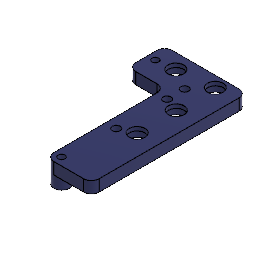
ZumoButtonAdapter (Autodesk Fusion 360 design; units mm, degrees)
Autodesk Fusion 360 part; units mm, degrees
sketch "Sketch1" plane through (17.2307, 33.6297, 85.118) normal (0, 0, 1) x (-0.000239, -1, 0)
  line L0 (5.7619, -33.0186) -> (14.2709, -33.0166)
  line L1 (14.2709, -33.0166) -> (14.2707, -32.1784)
  arc A0 (15.0833, -31.3654) -> (14.2707, -32.1784) centre (15.0835, -32.1782) ccw
  line L2 (15.0833, -31.3654) -> (20.4427, -31.3641)
  arc A1 (21.2557, -32.1767) -> (20.4427, -31.3641) centre (20.4429, -32.1769) ccw
  line L3 (21.2557, -32.1767) -> (21.2559, -33.0149)
  line L4 (21.2559, -33.0149) -> (36.4451, -33.0113)
  arc A2 (36.4451, -33.0113) -> (37.2577, -32.1983) centre (36.4449, -32.1985) ccw
  line L5 (37.2577, -32.1983) -> (37.2544, -18.2791)
  line L6 (37.2544, -18.2791) -> (35.9841, -17.0094)
  line L7 (35.9841, -17.0094) -> (35.9813, -5.3254)
  line L8 (35.9813, -5.3254) -> (37.251, -4.0551)
  line L9 (37.251, -4.0551) -> (37.249, 4.0729)
  line L10 (37.249, 4.0729) -> (35.4706, 5.8505)
  line L11 (35.4706, 5.8505) -> (35.4684, 14.9945)
  line L12 (35.4684, 14.9945) -> (37.246, 16.7729)
  line L13 (37.246, 16.7729) -> (37.2423, 32.2161)
  arc A3 (37.2423, 32.2161) -> (36.4293, 33.0287) centre (36.4295, 32.2159) ccw
  line L14 (36.4293, 33.0287) -> (21.2401, 33.0251)
  line L15 (21.2401, 33.0251) -> (21.2403, 32.1869)
  arc A4 (20.4277, 31.3739) -> (21.2403, 32.1869) centre (20.4275, 32.1867) ccw
  line L16 (20.4277, 31.3739) -> (15.0683, 31.3726)
  arc A5 (14.2553, 32.1852) -> (15.0683, 31.3726) centre (15.0681, 32.1854) ccw
  line L17 (14.2553, 32.1852) -> (14.2551, 33.0234)
  line L18 (14.2551, 33.0234) -> (5.7461, 33.0214)
  arc A6 (-0.6054, 39.3699) -> (5.7461, 33.0214) centre (5.7446, 39.3714) ccw
  line L19 (-0.6054, 39.3699) -> (-0.6071, 46.1771)
  arc A7 (-0.6071, 46.1771) -> (-1.4201, 46.9897) centre (-1.4199, 46.1769) ccw
  line L20 (-1.4201, 46.9897) -> (-11.2245, 46.9873)
  arc A8 (-11.2245, 46.9873) -> (-12.0371, 46.1743) centre (-11.2243, 46.1745) ccw
  line L21 (-12.0371, 46.1743) -> (-12.0354, 39.3671)
  arc A9 (-18.3839, 33.0156) -> (-12.0354, 39.3671) centre (-18.3854, 39.3656) ccw
  line L22 (-18.3839, 33.0156) -> (-22.0161, 33.0147)
  arc A10 (-22.8291, 33.8273) -> (-22.0161, 33.0147) centre (-22.0163, 33.8275) ccw
  line L23 (-22.8291, 33.8273) -> (-22.8302, 38.6025)
  line L24 (-22.8302, 38.6025) -> (-37.6892, 38.599)
  line L25 (-37.6892, 38.599) -> (-37.6881, 33.8238)
  arc A11 (-38.5007, 33.0108) -> (-37.6881, 33.8238) centre (-38.5009, 33.8236) ccw
  line L26 (-38.5007, 33.0108) -> (-44.7491, 33.0093)
  arc A12 (-44.7491, 33.0093) -> (-45.5617, 32.1963) centre (-44.7489, 32.1965) ccw
  line L27 (-45.5617, 32.1963) -> (-45.5463, -32.2181)
  arc A13 (-45.5463, -32.2181) -> (-44.7333, -33.0307) centre (-44.7335, -32.2179) ccw
  line L28 (-44.7333, -33.0307) -> (-38.4849, -33.0292)
  arc A14 (-37.6719, -33.8418) -> (-38.4849, -33.0292) centre (-38.4847, -33.842) ccw
  line L29 (-37.6719, -33.8418) -> (-37.6708, -38.617)
  line L30 (-37.6708, -38.617) -> (-22.8118, -38.6135)
  line L31 (-22.8118, -38.6135) -> (-22.8129, -33.8383)
  arc A15 (-22.0003, -33.0253) -> (-22.8129, -33.8383) centre (-22.0001, -33.8381) ccw
  line L32 (-22.0003, -33.0253) -> (-18.3681, -33.0244)
  arc A16 (-12.0166, -39.3729) -> (-18.3681, -33.0244) centre (-18.3666, -39.3744) ccw
  line L33 (-12.0166, -39.3729) -> (-12.0149, -46.1801)
  arc A17 (-12.0149, -46.1801) -> (-11.2019, -46.9927) centre (-11.2021, -46.1799) ccw
  line L34 (-11.2019, -46.9927) -> (-1.3975, -46.9903)
  arc A18 (-1.3975, -46.9903) -> (-0.5849, -46.1773) centre (-1.3977, -46.1775) ccw
  line L35 (-0.5849, -46.1773) -> (-0.5866, -39.3701)
  arc A19 (5.7619, -33.0186) -> (-0.5866, -39.3701) centre (5.7634, -39.3686) ccw
  circle A20 centre (23.7464, 15.0057) radius 1.0922
  arc A21 (33.2479, -24.524) -> (34.2639, -24.5238) centre (33.7559, -24.5239) ccw
  line L36 (33.2479, -24.524) -> (33.2469, -20.46)
  arc A22 (34.2629, -20.4598) -> (33.2469, -20.46) centre (33.7549, -20.4599) ccw
  line L37 (34.2629, -20.4598) -> (34.2639, -24.5238)
  line L38 (17.3197, -11.3359) -> (18.0697, -11.3357)
  line L39 (18.0697, -11.3357) -> (18.0697, -11.3457)
  line L40 (18.0697, -11.3457) -> (17.3197, -11.3459)
  line L41 (17.3197, -11.3459) -> (17.3197, -11.3359)
  line L42 (10.2071, -8.7236) -> (10.2071, -8.7135)
  line L43 (10.2071, -8.7135) -> (10.9571, -8.7133)
  line L44 (10.9571, -8.7133) -> (10.9571, -8.7234)
  line L45 (10.9571, -8.7234) -> (10.2071, -8.7236)
  line L46 (10.2052, -0.9336) -> (10.2052, -0.9236)
  line L47 (10.2052, -0.9236) -> (10.9552, -0.9234)
  line L48 (10.9552, -0.9234) -> (10.9552, -0.9334)
  line L49 (10.9552, -0.9334) -> (10.2052, -0.9336)
  line L50 (15.535, 28.7227) -> (16.1851, 28.7229)
  line L51 (16.1851, 28.7229) -> (16.185, 29.1979)
  line L52 (16.185, 29.1979) -> (15.635, 29.1977)
  line L53 (15.635, 29.1977) -> (15.6349, 29.7477)
  line L54 (15.6349, 29.7477) -> (19.7349, 29.7487)
  line L55 (19.7349, 29.7487) -> (19.735, 29.1987)
  line L56 (19.735, 29.1987) -> (19.185, 29.1986)
  line L57 (19.185, 29.1986) -> (19.1851, 28.7236)
  line L58 (19.1851, 28.7236) -> (19.8353, 28.7237)
  line L59 (19.8353, 28.7237) -> (19.8355, 27.6737)
  line L60 (19.8355, 27.6737) -> (19.1854, 27.6736)
  line L61 (19.1854, 27.6736) -> (19.1855, 27.1986)
  line L62 (19.1855, 27.1986) -> (19.7355, 27.1987)
  line L63 (19.7355, 27.1987) -> (19.7356, 26.6487)
  line L64 (19.7356, 26.6487) -> (15.6356, 26.6477)
  line L65 (15.6356, 26.6477) -> (15.6355, 27.1977)
  line L66 (15.6355, 27.1977) -> (16.1855, 27.1979)
  line L67 (16.1855, 27.1979) -> (16.1854, 27.6729)
  line L68 (16.1854, 27.6729) -> (15.5352, 27.6727)
  line L69 (15.5352, 27.6727) -> (15.535, 28.7227)
  line L70 (27.0977, 4.5955) -> (27.7479, 4.5956)
  line L71 (27.7479, 4.5956) -> (27.7478, 5.0706)
  line L72 (27.7478, 5.0706) -> (27.1978, 5.0705)
  line L73 (27.1978, 5.0705) -> (27.1977, 5.6205)
  line L74 (27.1977, 5.6205) -> (31.2977, 5.6215)
  line L75 (31.2977, 5.6215) -> (31.2978, 5.0715)
  line L76 (31.2978, 5.0715) -> (30.7478, 5.0714)
  line L77 (30.7478, 5.0714) -> (30.7479, 4.5964)
  line L78 (30.7479, 4.5964) -> (31.3981, 4.5965)
  line L79 (31.3981, 4.5965) -> (31.3983, 3.5465)
  line L80 (31.3983, 3.5465) -> (30.7481, 3.5464)
  line L81 (30.7481, 3.5464) -> (30.7483, 3.0714)
  line L82 (30.7483, 3.0714) -> (31.2983, 3.0715)
  line L83 (31.2983, 3.0715) -> (31.2984, 2.5215)
  line L84 (31.2984, 2.5215) -> (27.1984, 2.5205)
  line L85 (27.1984, 2.5205) -> (27.1983, 3.0705)
  line L86 (27.1983, 3.0705) -> (27.7483, 3.0706)
  line L87 (27.7483, 3.0706) -> (27.7481, 3.5456)
  line L88 (27.7481, 3.5456) -> (27.098, 3.5455)
  line L89 (27.098, 3.5455) -> (27.0977, 4.5955)
  line L90 (34.7063, 7.0473) -> (34.7064, 6.7973)
  line L91 (34.7064, 6.7973) -> (34.6513, 6.7973)
  arc A23 (34.4064, 6.6472) -> (34.6513, 6.7973) centre (34.4063, 6.9222) ccw
  line L92 (34.4064, 6.6472) -> (33.8064, 6.6471)
  arc A24 (33.8063, 7.1971) -> (33.8064, 6.6471) centre (33.8063, 6.9221) ccw
  line L93 (33.8063, 7.1971) -> (34.4063, 7.1972)
  arc A25 (34.6513, 7.0473) -> (34.4063, 7.1972) centre (34.4063, 6.9222) ccw
  line L94 (34.6513, 7.0473) -> (34.7063, 7.0473)
  line L95 (-7.8006, -43.5709) -> (-4.8006, -43.5702)
  line L96 (-4.8006, -43.5702) -> (-4.8003, -44.5702)
  line L97 (-4.8003, -44.5702) -> (-5.3003, -44.5703)
  line L98 (-5.3003, -44.5703) -> (-5.3003, -44.7203)
  arc A26 (-6.1501, -45.5705) -> (-5.3003, -44.7203) centre (-6.1503, -44.7205) ccw
  line L99 (-6.1501, -45.5705) -> (-6.4501, -45.5706)
  arc A27 (-7.3003, -44.7208) -> (-6.4501, -45.5706) centre (-6.4503, -44.7206) ccw
  line L100 (-7.3003, -44.7208) -> (-7.3003, -44.5708)
  line L101 (-7.3003, -44.5708) -> (-7.8003, -44.5709)
  line L102 (-7.8003, -44.5709) -> (-7.8006, -43.5709)
  line L103 (-4.8214, 43.5678) -> (-7.8214, 43.5671)
  line L104 (-7.8214, 43.5671) -> (-7.8217, 44.5671)
  line L105 (-7.8217, 44.5671) -> (-7.3217, 44.5672)
  line L106 (-7.3217, 44.5672) -> (-7.3217, 44.7172)
  arc A28 (-6.4719, 45.5674) -> (-7.3217, 44.7172) centre (-6.4717, 44.7174) ccw
  line L107 (-6.4719, 45.5674) -> (-6.1719, 45.5675)
  arc A29 (-5.3217, 44.7177) -> (-6.1719, 45.5675) centre (-6.1717, 44.7175) ccw
  line L108 (-5.3217, 44.7177) -> (-5.3217, 44.5677)
  line L109 (-5.3217, 44.5677) -> (-4.8217, 44.5678)
  line L110 (-4.8217, 44.5678) -> (-4.8214, 43.5678)
  line L111 (-20.9261, 8.615) -> (-20.9262, 9.01)
  line L112 (-20.9262, 9.01) -> (-16.8462, 9.011)
  line L113 (-16.8462, 9.011) -> (-16.8461, 8.616)
  line L114 (-16.8461, 8.616) -> (-20.9261, 8.615)
  line L115 (-20.1809, 8.0152) -> (-20.1807, 7.2152)
  line L116 (-20.1807, 7.2152) -> (-21.6857, 7.2148)
  line L117 (-21.6857, 7.2148) -> (-21.8858, 7.4148)
  line L118 (-21.8858, 7.4148) -> (-21.8859, 7.8148)
  line L119 (-21.8859, 7.8148) -> (-21.6859, 8.0148)
  line L120 (-21.6859, 8.0148) -> (-20.1809, 8.0152)
  line L121 (-20.9255, 6.075) -> (-20.9256, 6.615)
  line L122 (-20.9256, 6.615) -> (-16.8456, 6.616)
  line L123 (-16.8456, 6.616) -> (-16.8455, 6.076)
  line L124 (-16.8455, 6.076) -> (-20.9255, 6.075)
  line L125 (-16.8419, -8.624) -> (-16.8418, -9.019)
  line L126 (-16.8418, -9.019) -> (-20.9218, -9.02)
  line L127 (-20.9218, -9.02) -> (-20.9219, -8.625)
  line L128 (-20.9219, -8.625) -> (-16.8419, -8.624)
  line L129 (-20.9249, 3.535) -> (-20.925, 4.075)
  line L130 (-20.925, 4.075) -> (-16.845, 4.076)
  line L131 (-16.845, 4.076) -> (-16.8449, 3.536)
  line L132 (-16.8449, 3.536) -> (-20.9249, 3.535)
  line L133 (-15.8858, 7.4162) -> (-16.0857, 7.2161)
  line L134 (-16.0857, 7.2161) -> (-17.5907, 7.2158)
  line L135 (-17.5907, 7.2158) -> (-17.5909, 8.0158)
  line L136 (-17.5909, 8.0158) -> (-16.0859, 8.0161)
  line L137 (-16.0859, 8.0161) -> (-15.8859, 7.8162)
  line L138 (-15.8859, 7.8162) -> (-15.8858, 7.4162)
  line L139 (-15.8852, 4.8762) -> (-16.0851, 4.6761)
  line L140 (-16.0851, 4.6761) -> (-17.5901, 4.6758)
  line L141 (-17.5901, 4.6758) -> (-17.5903, 5.4758)
  line L142 (-17.5903, 5.4758) -> (-16.0853, 5.4761)
  line L143 (-16.0853, 5.4761) -> (-15.8853, 5.2762)
  line L144 (-15.8853, 5.2762) -> (-15.8852, 4.8762)
  line L145 (-15.8846, 2.3362) -> (-16.0845, 2.1361)
  line L146 (-16.0845, 2.1361) -> (-17.5895, 2.1358)
  line L147 (-17.5895, 2.1358) -> (-17.5897, 2.9358)
  line L148 (-17.5897, 2.9358) -> (-16.0847, 2.9361)
  line L149 (-16.0847, 2.9361) -> (-15.8847, 2.7362)
  line L150 (-15.8847, 2.7362) -> (-15.8846, 2.3362)
  line L151 (-15.884, -0.2038) -> (-16.0839, -0.4039)
  line L152 (-16.0839, -0.4039) -> (-17.5889, -0.4042)
  line L153 (-17.5889, -0.4042) -> (-17.5891, 0.3958)
  line L154 (-17.5891, 0.3958) -> (-16.0841, 0.3961)
  line L155 (-16.0841, 0.3961) -> (-15.8841, 0.1962)
  line L156 (-15.8841, 0.1962) -> (-15.884, -0.2038)
  line L157 (-15.8833, -2.7438) -> (-16.0833, -2.9439)
  line L158 (-16.0833, -2.9439) -> (-17.5883, -2.9442)
  line L159 (-17.5883, -2.9442) -> (-17.5885, -2.1442)
  line L160 (-17.5885, -2.1442) -> (-16.0835, -2.1439)
  line L161 (-16.0835, -2.1439) -> (-15.8834, -2.3438)
  line L162 (-15.8834, -2.3438) -> (-15.8833, -2.7438)
  line L163 (-15.8827, -5.2838) -> (-16.0827, -5.4839)
  line L164 (-16.0827, -5.4839) -> (-17.5877, -5.4842)
  line L165 (-17.5877, -5.4842) -> (-17.5879, -4.6842)
  line L166 (-17.5879, -4.6842) -> (-16.0829, -4.6839)
  line L167 (-16.0829, -4.6839) -> (-15.8828, -4.8838)
  line L168 (-15.8828, -4.8838) -> (-15.8827, -5.2838)
  line L169 (-15.8821, -7.8238) -> (-16.0821, -8.0239)
  line L170 (-16.0821, -8.0239) -> (-17.5871, -8.0242)
  line L171 (-17.5871, -8.0242) -> (-17.5873, -7.2242)
  line L172 (-17.5873, -7.2242) -> (-16.0823, -7.2239)
  line L173 (-16.0823, -7.2239) -> (-15.8822, -7.4238)
  line L174 (-15.8822, -7.4238) -> (-15.8821, -7.8238)
  line L175 (-20.1803, 5.4752) -> (-20.1801, 4.6752)
  line L176 (-20.1801, 4.6752) -> (-21.6851, 4.6748)
  line L177 (-21.6851, 4.6748) -> (-21.8852, 4.8748)
  line L178 (-21.8852, 4.8748) -> (-21.8853, 5.2748)
  line L179 (-21.8853, 5.2748) -> (-21.6853, 5.4748)
  line L180 (-21.6853, 5.4748) -> (-20.1803, 5.4752)
  line L181 (-20.1797, 2.9352) -> (-20.1795, 2.1352)
  line L182 (-20.1795, 2.1352) -> (-21.6845, 2.1348)
  line L183 (-21.6845, 2.1348) -> (-21.8846, 2.3348)
  line L184 (-21.8846, 2.3348) -> (-21.8847, 2.7348)
  line L185 (-21.8847, 2.7348) -> (-21.6847, 2.9348)
  line L186 (-21.6847, 2.9348) -> (-20.1797, 2.9352)
  line L187 (-20.1791, 0.3952) -> (-20.1789, -0.4048)
  line L188 (-20.1789, -0.4048) -> (-21.6839, -0.4052)
  line L189 (-21.6839, -0.4052) -> (-21.884, -0.2052)
  line L190 (-21.884, -0.2052) -> (-21.8841, 0.1948)
  line L191 (-21.8841, 0.1948) -> (-21.6841, 0.3948)
  line L192 (-21.6841, 0.3948) -> (-20.1791, 0.3952)
  line L193 (-20.1785, -2.1448) -> (-20.1783, -2.9448)
  line L194 (-20.1783, -2.9448) -> (-21.6833, -2.9452)
  line L195 (-21.6833, -2.9452) -> (-21.8833, -2.7452)
  line L196 (-21.8833, -2.7452) -> (-21.8834, -2.3452)
  line L197 (-21.8834, -2.3452) -> (-21.6835, -2.1452)
  line L198 (-21.6835, -2.1452) -> (-20.1785, -2.1448)
  line L199 (-20.1779, -4.6848) -> (-20.1777, -5.4848)
  line L200 (-20.1777, -5.4848) -> (-21.6827, -5.4852)
  line L201 (-21.6827, -5.4852) -> (-21.8827, -5.2852)
  line L202 (-21.8827, -5.2852) -> (-21.8828, -4.8852)
  line L203 (-21.8828, -4.8852) -> (-21.6829, -4.6852)
  line L204 (-21.6829, -4.6852) -> (-20.1779, -4.6848)
  line L205 (-20.1773, -7.2248) -> (-20.1771, -8.0248)
  line L206 (-20.1771, -8.0248) -> (-21.6821, -8.0252)
  line L207 (-21.6821, -8.0252) -> (-21.8821, -7.8252)
  line L208 (-21.8821, -7.8252) -> (-21.8822, -7.4252)
  line L209 (-21.8822, -7.4252) -> (-21.6823, -7.2252)
  line L210 (-21.6823, -7.2252) -> (-20.1773, -7.2248)
  circle A30 centre (-39.244, -25.0094) radius 1.0922
  circle A31 centre (-12.2566, 27.4971) radius 1.0922
  circle A32 centre (-12.2434, -27.5029) radius 1.0922
  circle A33 centre (-39.256, 24.9906) radius 1.0922
  circle A34 centre (-12.25, -0.0029) radius 1.0922
  circle A35 centre (23.7434, 27.5057) radius 1.0922
  circle A36 centre (11.7434, 27.5028) radius 1.0922
  circle A37 centre (11.7566, -27.4972) radius 1.0922
  circle A38 centre (23.7566, -27.4943) radius 1.0922
  circle A39 centre (-6.8132, -24.1316) radius 0.508
  circle A40 centre (-4.2732, -24.131) radius 0.508
  circle A41 centre (-1.7332, -24.1304) radius 0.508
  circle A42 centre (10.9668, -24.1274) radius 0.508
  circle A43 centre (13.5068, -24.1268) radius 0.508
  circle A44 centre (16.0468, -24.1262) radius 0.508
  circle A45 centre (18.5862, -21.5856) radius 0.508
  circle A46 centre (8.4262, -21.588) radius 0.508
  circle A47 centre (5.8868, -24.1286) radius 0.508
  circle A48 centre (8.4268, -24.128) radius 0.508
  circle A49 centre (18.5868, -24.1256) radius 0.508
  circle A50 centre (-34.003, 12.6919) radius 0.508
  circle A51 centre (3.3468, -24.1292) radius 0.508
  circle A52 centre (0.8068, -24.1298) radius 0.508
  circle A53 centre (-11.8932, -24.1329) radius 0.508
  circle A54 centre (-9.3532, -24.1322) radius 0.508
  circle A55 centre (-11.9042, 21.5871) radius 0.508
  circle A56 centre (0.7958, 21.5902) radius 0.508
  circle A57 centre (3.3358, 21.5908) radius 0.508
  circle A58 centre (5.8758, 21.5914) radius 0.508
  circle A59 centre (8.4158, 21.592) radius 0.508
  circle A60 centre (18.5758, 21.5944) radius 0.508
  circle A61 centre (16.0462, -21.5862) radius 0.508
  circle A62 centre (13.5062, -21.5868) radius 0.508
  circle A63 centre (10.9662, -21.5874) radius 0.508
  circle A64 centre (5.8862, -21.5886) radius 0.508
  circle A65 centre (3.3462, -21.5892) radius 0.508
  circle A66 centre (0.8062, -21.5898) radius 0.508
  circle A67 centre (-11.8938, -21.5929) radius 0.508
  circle A68 centre (-9.3538, -21.5922) radius 0.508
  circle A69 centre (-6.8138, -21.5916) radius 0.508
  circle A70 centre (-4.2738, -21.591) radius 0.508
  circle A71 centre (-1.7338, -21.5904) radius 0.508
  circle A72 centre (-44.2825, -6.3606) radius 0.508
  circle A73 centre (-44.2819, -8.9006) radius 0.508
  circle A74 centre (-44.2764, -31.7606) radius 0.508
  circle A75 centre (-41.7364, -31.76) radius 0.508
  circle A76 centre (-5.0317, -38.8632) radius 0.508
  circle A77 centre (-7.5717, -38.8638) radius 0.508
  circle A78 centre (-5.0311, -41.4032) radius 0.508
  circle A79 centre (-7.5711, -41.4038) radius 0.508
  circle A80 centre (-7.5903, 38.8602) radius 0.508
  circle A81 centre (-5.0503, 38.8608) radius 0.508
  circle A82 centre (-7.5909, 41.4002) radius 0.508
  circle A83 centre (-5.0509, 41.4008) radius 0.508
  circle A84 centre (-1.2226, -35.0523) radius 0.508
  circle A85 centre (-1.2394, 35.0517) radius 0.508
  circle A86 centre (-44.2843, 1.2594) radius 0.508
  circle A87 centre (-44.2837, -1.2806) radius 0.508
  circle A88 centre (-44.2813, -11.4406) radius 0.508
  circle A89 centre (-44.2807, -13.9806) radius 0.508
  circle A90 centre (-44.28, -16.5206) radius 0.508
  circle A91 centre (-44.2794, -19.0606) radius 0.508
  circle A92 centre (-26.503, 12.6936) radius 0.508
  circle A93 centre (-33.997, -12.7081) radius 0.508
  circle A94 centre (-26.4969, -12.7064) radius 0.508
  circle A95 centre (-44.2831, -3.8206) radius 0.508
  circle A96 centre (-44.2861, 8.8794) radius 0.508
  circle A97 centre (-44.2867, 11.4194) radius 0.508
  circle A98 centre (-44.2873, 13.9594) radius 0.508
  circle A99 centre (-44.288, 16.4994) radius 0.508
  circle A100 centre (-44.2886, 19.0394) radius 0.508
  circle A101 centre (-44.2855, 6.3394) radius 0.508
  circle A102 centre (-44.2849, 3.7994) radius 0.508
  circle A103 centre (-39.2049, 3.8006) radius 0.508
  circle A104 centre (-39.2055, 6.3406) radius 0.508
  circle A105 centre (-39.2061, 8.8806) radius 0.508
  circle A106 centre (-39.2067, 11.4206) radius 0.508
  circle A107 centre (-39.2073, 13.9606) radius 0.508
  circle A108 centre (-39.2043, 1.2606) radius 0.508
  circle A109 centre (-39.2037, -1.2794) radius 0.508
  circle A110 centre (-39.2031, -3.8194) radius 0.508
  circle A111 centre (-39.2025, -6.3594) radius 0.508
  circle A112 centre (-41.7425, -6.36) radius 0.508
  circle A113 centre (-39.2007, -13.9794) radius 0.508
  circle A114 centre (-39.2013, -11.4394) radius 0.508
  circle A115 centre (-39.2019, -8.8994) radius 0.508
  circle A116 centre (-41.7431, -3.82) radius 0.508
  circle A117 centre (-41.7437, -1.28) radius 0.508
  circle A118 centre (-41.7443, 1.26) radius 0.508
  circle A119 centre (-41.7473, 13.96) radius 0.508
  line L211 (-6.9445, -6.4152) -> (-7.1985, -6.4152)
  arc A120 (-7.1987, -5.5262) -> (-7.1985, -6.4152) centre (-7.1986, -5.9707) ccw
  line L212 (-7.1987, -5.5262) -> (-6.9447, -5.5262)
  arc A121 (-6.9445, -6.4152) -> (-6.9447, -5.5262) centre (-6.9446, -5.9707) ccw
  line L213 (-3.4527, -5.5253) -> (-3.1987, -5.5253)
  arc A122 (-3.1985, -6.4143) -> (-3.1987, -5.5253) centre (-3.1986, -5.9698) ccw
  line L214 (-3.1985, -6.4143) -> (-3.4525, -6.4143)
  arc A123 (-3.4527, -5.5253) -> (-3.4525, -6.4143) centre (-3.4526, -5.9698) ccw
  circle A124 centre (-41.7516, 31.74) radius 0.508
  circle A125 centre (-44.2916, 31.7394) radius 0.508
  line L215 (34.2521, 24.5402) -> (34.2531, 20.4762)
  arc A126 (33.2371, 20.476) -> (34.2531, 20.4762) centre (33.7451, 20.4761) ccw
  line L216 (33.2371, 20.476) -> (33.2361, 24.54)
  arc A127 (34.2521, 24.5402) -> (33.2361, 24.54) centre (33.7441, 24.5401) ccw
  circle A128 centre (-4.2848, 24.129) radius 0.508
  circle A129 centre (-6.8248, 24.1284) radius 0.508
  circle A130 centre (-9.3648, 24.1278) radius 0.508
  circle A131 centre (-11.9048, 24.1271) radius 0.508
  circle A132 centre (0.7952, 24.1302) radius 0.508
  circle A133 centre (3.3352, 24.1308) radius 0.508
  circle A134 centre (5.8752, 24.1314) radius 0.508
  circle A135 centre (8.4152, 24.132) radius 0.508
  circle A136 centre (18.5752, 24.1344) radius 0.508
  circle A137 centre (16.0358, 21.5938) radius 0.508
  circle A138 centre (13.4958, 21.5932) radius 0.508
  circle A139 centre (10.9558, 21.5926) radius 0.508
  circle A140 centre (-1.7442, 21.5896) radius 0.508
  circle A141 centre (-4.2842, 21.589) radius 0.508
  circle A142 centre (-6.8242, 21.5884) radius 0.508
  circle A143 centre (-9.3642, 21.5878) radius 0.508
  circle A144 centre (-6.3194, 35.0505) radius 0.508
  circle A145 centre (-8.8594, 35.0499) radius 0.508
  circle A146 centre (-41.7407, -13.98) radius 0.508
  circle A147 centre (-41.7413, -11.44) radius 0.508
  circle A148 centre (-41.7419, -8.9) radius 0.508
  circle A149 centre (-41.7449, 3.8) radius 0.508
  circle A150 centre (-41.7455, 6.34) radius 0.508
  circle A151 centre (-41.7461, 8.88) radius 0.508
  circle A152 centre (-41.7467, 11.42) radius 0.508
  circle A153 centre (-3.7626, -35.0529) radius 0.508
  circle A154 centre (-6.3026, -35.0535) radius 0.508
  circle A155 centre (-8.8426, -35.0541) radius 0.508
  circle A156 centre (-3.7794, 35.0511) radius 0.508
  circle A157 centre (16.0352, 24.1338) radius 0.508
  circle A158 centre (13.4952, 24.1332) radius 0.508
  circle A159 centre (10.9552, 24.1326) radius 0.508
  circle A160 centre (-1.7448, 24.1296) radius 0.508
  line L217 (-18.8814, -25.5025) -> (-19.2064, -25.5026)
  arc A161 (-19.2814, -25.4276) -> (-19.2064, -25.5026) centre (-19.2064, -25.4276) ccw
  line L218 (-19.2814, -25.4276) -> (-19.2821, -22.4776)
  arc A162 (-19.2071, -22.4026) -> (-19.2821, -22.4776) centre (-19.2071, -22.4776) ccw
  line L219 (-19.2071, -22.4026) -> (-18.1321, -22.4023)
  line L220 (-18.1321, -22.4023) -> (-18.1321, -22.3923)
  line L221 (-18.1321, -22.3923) -> (-17.3321, -22.3922)
  line L222 (-17.3321, -22.3922) -> (-17.3321, -22.4022)
  line L223 (-17.3321, -22.4022) -> (-16.2571, -22.4019)
  arc A163 (-16.1821, -22.4769) -> (-16.2571, -22.4019) centre (-16.2571, -22.4769) ccw
  line L224 (-16.1821, -22.4769) -> (-16.1814, -25.4269)
  arc A164 (-16.2564, -25.5019) -> (-16.1814, -25.4269) centre (-16.2564, -25.4269) ccw
  line L225 (-16.2564, -25.5019) -> (-16.5814, -25.502)
  line L226 (-16.5814, -25.502) -> (-16.5814, -25.512)
  line L227 (-16.5814, -25.512) -> (-17.1314, -25.5121)
  line L228 (-17.1314, -25.5121) -> (-17.1314, -25.5021)
  line L229 (-17.1314, -25.5021) -> (-18.3314, -25.5024)
  line L230 (-18.3314, -25.5024) -> (-18.3314, -25.5124)
  line L231 (-18.3314, -25.5124) -> (-18.8814, -25.5125)
  line L232 (-18.8814, -25.5125) -> (-18.8814, -25.5025)
  line L233 (-16.8442, 0.996) -> (-20.9242, 0.995)
  line L234 (-20.9242, 0.995) -> (-20.9244, 1.535)
  line L235 (-20.9244, 1.535) -> (-16.8444, 1.536)
  line L236 (-16.8444, 1.536) -> (-16.8442, 0.996)
  line L237 (-16.8436, -1.544) -> (-20.9236, -1.545)
  line L238 (-20.9236, -1.545) -> (-20.9238, -1.005)
  line L239 (-20.9238, -1.005) -> (-16.8438, -1.004)
  line L240 (-16.8438, -1.004) -> (-16.8436, -1.544)
  line L241 (-16.843, -4.084) -> (-20.923, -4.085)
  line L242 (-20.923, -4.085) -> (-20.9232, -3.545)
  line L243 (-20.9232, -3.545) -> (-16.8432, -3.544)
  line L244 (-16.8432, -3.544) -> (-16.843, -4.084)
  line L245 (-16.8424, -6.624) -> (-20.9224, -6.625)
  line L246 (-20.9224, -6.625) -> (-20.9225, -6.085)
  line L247 (-20.9225, -6.085) -> (-16.8425, -6.084)
  line L248 (-16.8425, -6.084) -> (-16.8424, -6.624)
  line L249 (34.6496, 14.0473) -> (34.7046, 14.0473)
  line L250 (34.7046, 14.0473) -> (34.7047, 13.7973)
  line L251 (34.7047, 13.7973) -> (34.6496, 13.7973)
  arc A165 (34.4047, 13.6472) -> (34.6496, 13.7973) centre (34.4047, 13.9222) ccw
  line L252 (34.4047, 13.6472) -> (33.8047, 13.6471)
  arc A166 (33.8046, 14.1971) -> (33.8047, 13.6471) centre (33.8047, 13.9221) ccw
  line L253 (33.8046, 14.1971) -> (34.4046, 14.1972)
  arc A167 (34.6496, 14.0473) -> (34.4046, 14.1972) centre (34.4047, 13.9222) ccw
  line L254 (31.656, 8.2216) -> (31.656, 8.1862)
  arc A168 (31.6811, 8.0716) -> (31.656, 8.1862) centre (31.4061, 8.0715) ccw
  line L255 (31.6811, 8.0716) -> (31.6811, 7.7716)
  arc A169 (31.6562, 7.657) -> (31.6811, 7.7716) centre (31.4061, 7.7715) ccw
  line L256 (31.6562, 7.657) -> (31.6562, 7.6216)
  line L257 (31.6562, 7.6216) -> (31.6367, 7.6216)
  arc A170 (31.1311, 7.7715) -> (31.6367, 7.6216) centre (31.4061, 7.7715) ccw
  line L258 (31.1311, 7.7715) -> (31.1311, 8.0715)
  arc A171 (31.6365, 8.2216) -> (31.1311, 8.0715) centre (31.4061, 8.0715) ccw
  line L259 (31.6365, 8.2216) -> (31.656, 8.2216)
  line L260 (31.655, 12.657) -> (31.655, 12.6216)
  line L261 (31.655, 12.6216) -> (31.6355, 12.6216)
  arc A172 (31.1299, 12.7714) -> (31.6355, 12.6216) centre (31.4049, 12.7715) ccw
  line L262 (31.1299, 12.7714) -> (31.1299, 13.0714)
  arc A173 (31.6353, 13.2216) -> (31.1299, 13.0714) centre (31.4049, 13.0715) ccw
  line L263 (31.6353, 13.2216) -> (31.6548, 13.2216)
  line L264 (31.6548, 13.2216) -> (31.6548, 13.1861)
  arc A174 (31.6799, 13.0716) -> (31.6548, 13.1861) centre (31.4049, 13.0715) ccw
  line L265 (31.6799, 13.0716) -> (31.6799, 12.7716)
  arc A175 (31.655, 12.657) -> (31.6799, 12.7716) centre (31.4049, 12.7715) ccw
  line L266 (34.9768, -7.3176) -> (35.3768, -7.3175)
  line L267 (35.3768, -7.3175) -> (35.3769, -7.8425)
  line L268 (35.3769, -7.8425) -> (35.3785, -14.4925)
  line L269 (35.3785, -14.4925) -> (35.3786, -15.0175)
  line L270 (35.3786, -15.0175) -> (34.9786, -15.0176)
  line L271 (34.9786, -15.0176) -> (34.9785, -14.5176)
  line L272 (34.9785, -14.5176) -> (33.1785, -14.5181)
  line L273 (33.1785, -14.5181) -> (33.1786, -15.0181)
  line L274 (33.1786, -15.0181) -> (32.7786, -15.0182)
  line L275 (32.7786, -15.0182) -> (32.7785, -14.4932)
  line L276 (32.7785, -14.4932) -> (32.7783, -13.6182)
  line L277 (32.7783, -13.6182) -> (31.8783, -13.6184)
  line L278 (31.8783, -13.6184) -> (31.8782, -13.2184)
  line L279 (31.8782, -13.2184) -> (32.7782, -13.2182)
  line L280 (32.7782, -13.2182) -> (32.7775, -10.6182)
  line L281 (32.7775, -10.6182) -> (31.8775, -10.6184)
  line L282 (31.8775, -10.6184) -> (31.8774, -10.2184)
  line L283 (31.8774, -10.2184) -> (32.7774, -10.2182)
  line L284 (32.7774, -10.2182) -> (32.7772, -9.1182)
  line L285 (32.7772, -9.1182) -> (31.8772, -9.1184)
  line L286 (31.8772, -9.1184) -> (31.8771, -8.7184)
  line L287 (31.8771, -8.7184) -> (32.7771, -8.7182)
  line L288 (32.7771, -8.7182) -> (32.7769, -7.8432)
  line L289 (32.7769, -7.8432) -> (32.7768, -7.3182)
  line L290 (32.7768, -7.3182) -> (33.1768, -7.3181)
  line L291 (33.1768, -7.3181) -> (33.1769, -7.8181)
  line L292 (33.1769, -7.8181) -> (34.9769, -7.8176)
  line L293 (34.9769, -7.8176) -> (34.9768, -7.3176)
  line L294 (27.0916, 29.9955) -> (27.7418, 29.9956)
  line L295 (27.7418, 29.9956) -> (27.7417, 30.4706)
  line L296 (27.7417, 30.4706) -> (27.1917, 30.4705)
  line L297 (27.1917, 30.4705) -> (27.1916, 31.0205)
  line L298 (27.1916, 31.0205) -> (31.2916, 31.0215)
  line L299 (31.2916, 31.0215) -> (31.2917, 30.4715)
  line L300 (31.2917, 30.4715) -> (30.7417, 30.4714)
  line L301 (30.7417, 30.4714) -> (30.7418, 29.9964)
  line L302 (30.7418, 29.9964) -> (31.392, 29.9965)
  line L303 (31.392, 29.9965) -> (31.3922, 28.9465)
  line L304 (31.3922, 28.9465) -> (30.7421, 28.9464)
  line L305 (30.7421, 28.9464) -> (30.7422, 28.4714)
  line L306 (30.7422, 28.4714) -> (31.2922, 28.4715)
  line L307 (31.2922, 28.4715) -> (31.2923, 27.9215)
  line L308 (31.2923, 27.9215) -> (27.1923, 27.9205)
  line L309 (27.1923, 27.9205) -> (27.1922, 28.4705)
  line L310 (27.1922, 28.4705) -> (27.7422, 28.4706)
  line L311 (27.7422, 28.4706) -> (27.7421, 28.9456)
  line L312 (27.7421, 28.9456) -> (27.0919, 28.9455)
  line L313 (27.0919, 28.9455) -> (27.0916, 29.9955)
  line L314 (27.0947, 17.2955) -> (27.7449, 17.2956)
  line L315 (27.7449, 17.2956) -> (27.7447, 17.7706)
  line L316 (27.7447, 17.7706) -> (27.1947, 17.7705)
  line L317 (27.1947, 17.7705) -> (27.1946, 18.3205)
  line L318 (27.1946, 18.3205) -> (31.2946, 18.3215)
  line L319 (31.2946, 18.3215) -> (31.2947, 17.7715)
  line L320 (31.2947, 17.7715) -> (30.7447, 17.7714)
  line L321 (30.7447, 17.7714) -> (30.7449, 17.2964)
  line L322 (30.7449, 17.2964) -> (31.395, 17.2965)
  line L323 (31.395, 17.2965) -> (31.3953, 16.2465)
  line L324 (31.3953, 16.2465) -> (30.7451, 16.2464)
  line L325 (30.7451, 16.2464) -> (30.7452, 15.7714)
  line L326 (30.7452, 15.7714) -> (31.2952, 15.7715)
  line L327 (31.2952, 15.7715) -> (31.2954, 15.2215)
  line L328 (31.2954, 15.2215) -> (27.1954, 15.2205)
  line L329 (27.1954, 15.2205) -> (27.1952, 15.7705)
  line L330 (27.1952, 15.7705) -> (27.7452, 15.7706)
  line L331 (27.7452, 15.7706) -> (27.7451, 16.2456)
  line L332 (27.7451, 16.2456) -> (27.0949, 16.2455)
  line L333 (27.0949, 16.2455) -> (27.0947, 17.2955)
  line L334 (26.963, -24.9655) -> (26.963, -24.9755)
  line L335 (26.963, -24.9755) -> (26.213, -24.9757)
  line L336 (26.213, -24.9757) -> (26.213, -24.9657)
  line L337 (26.213, -24.9657) -> (26.963, -24.9655)
  line L338 (26.9611, -17.1755) -> (26.9611, -17.1856)
  line L339 (26.9611, -17.1856) -> (26.2111, -17.1858)
  line L340 (26.2111, -17.1858) -> (26.2111, -17.1757)
  line L341 (26.2111, -17.1757) -> (26.9611, -17.1755)
  line L342 (17.3172, -0.9328) -> (17.3172, -0.9228)
  line L343 (17.3172, -0.9228) -> (18.0672, -0.9227)
  line L344 (18.0672, -0.9227) -> (18.0672, -0.9327)
  line L345 (18.0672, -0.9327) -> (17.3172, -0.9328)
  line L346 (17.3191, -8.7228) -> (17.3191, -8.7128)
  line L347 (17.3191, -8.7128) -> (18.0691, -8.7126)
  line L348 (18.0691, -8.7126) -> (18.0691, -8.7227)
  line L349 (18.0691, -8.7227) -> (17.3191, -8.7228)
  line L350 (-16.0892, 30.2032) -> (-16.3892, 30.2031)
  line L351 (-16.3892, 30.2031) -> (-16.3894, 31.0031)
  line L352 (-16.3894, 31.0031) -> (-16.0894, 31.0032)
  line L353 (-16.0894, 31.0032) -> (-16.0892, 30.2032)
  line L354 (-14.7894, 31.0035) -> (-14.7892, 30.2035)
  line L355 (-14.7892, 30.2035) -> (-15.0892, 30.2034)
  line L356 (-15.0892, 30.2034) -> (-15.0894, 31.0034)
  line L357 (-15.0894, 31.0034) -> (-14.7894, 31.0035)
  line L358 (-15.0748, -30.2107) -> (-14.7748, -30.2106)
  line L359 (-14.7748, -30.2106) -> (-14.7746, -31.0106)
  line L360 (-14.7746, -31.0106) -> (-15.0746, -31.0107)
  line L361 (-15.0746, -31.0107) -> (-15.0748, -30.2107)
  line L362 (-16.3746, -31.011) -> (-16.3748, -30.211)
  line L363 (-16.3748, -30.211) -> (-16.0748, -30.2109)
  line L364 (-16.0748, -30.2109) -> (-16.0746, -31.0109)
  line L365 (-16.0746, -31.0109) -> (-16.3746, -31.011)
  line L366 (24.1713, 23.7358) -> (23.8713, 23.7358)
  line L367 (23.8713, 23.7358) -> (23.8711, 24.5358)
  line L368 (23.8711, 24.5358) -> (24.1711, 24.5358)
  line L369 (24.1711, 24.5358) -> (24.1713, 23.7358)
  line L370 (25.4711, 24.5361) -> (25.4713, 23.7361)
  line L371 (25.4713, 23.7361) -> (25.1713, 23.7361)
  line L372 (25.1713, 23.7361) -> (25.1711, 24.5361)
  line L373 (25.1711, 24.5361) -> (25.4711, 24.5361)
  line L374 (24.1766, 1.5108) -> (23.8766, 1.5108)
  line L375 (23.8766, 1.5108) -> (23.8764, 2.3108)
  line L376 (23.8764, 2.3108) -> (24.1764, 2.3108)
  line L377 (24.1764, 2.3108) -> (24.1766, 1.5108)
  line L378 (25.4764, 2.3111) -> (25.4766, 1.5111)
  line L379 (25.4766, 1.5111) -> (25.1766, 1.5111)
  line L380 (25.1766, 1.5111) -> (25.1764, 2.3111)
  line L381 (25.1764, 2.3111) -> (25.4764, 2.3111)
  line L382 (24.1727, 18.0208) -> (23.8727, 18.0208)
  line L383 (23.8727, 18.0208) -> (23.8725, 18.8208)
  line L384 (23.8725, 18.8208) -> (24.1725, 18.8208)
  line L385 (24.1725, 18.8208) -> (24.1727, 18.0208)
  line L386 (25.4725, 18.8211) -> (25.4727, 18.0211)
  line L387 (25.4727, 18.0211) -> (25.1727, 18.0211)
  line L388 (25.1727, 18.0211) -> (25.1725, 18.8211)
  line L389 (25.1725, 18.8211) -> (25.4725, 18.8211)
  circle A176 centre (-0.2566, 27.4999) radius 1.0922
  circle A177 centre (23.7536, -14.9943) radius 1.0922
  circle A178 centre (-0.2434, -27.5001) radius 1.0922
ref_plane "WorkPlane1" through (17.2302, 37.7817, 97.818) normal (0, 0, 1) x (-0.000239, -1, 0)
sketch "Sketch2" plane through (-4.152, -0.0015, 97.818) normal (0, 0, 1) x (1, 0, 0)
  circle A0 centre (15.8954, 27.5043) radius 1.0922
  circle A1 centre (27.9056, -14.9928) radius 1.0922
  line L0 (21.2011, 28.6273) -> (20.7095, 28.6271) construction
  line L1 (20.7095, 28.6271) -> (20.7097, 27.7718) construction
  line L2 (20.7097, 27.7718) -> (21.2013, 27.7719) construction
  ellipse E0 centre (21.1985, 27.6699) end of major axis (21.2461, 27.761) minor radius 0.0993 (21.2759, 27.7368) -> (21.2013, 27.7719) ccw
  arc A2 (21.2759, 27.7368) -> (22.3989, 27.7371) centre (21.8372, 28.1997) ccw construction
  ellipse E1 centre (22.4758, 27.67) end of major axis (22.4358, 27.7647) minor radius 0.0993 (22.4734, 27.7722) -> (22.3989, 27.7371) ccw
  line L3 (22.4734, 27.7722) -> (22.965, 27.7724) construction
  line L4 (22.965, 27.7724) -> (22.9648, 28.6277) construction
  line L5 (22.9648, 28.6277) -> (22.4259, 28.6275) construction
  arc A3 (22.4259, 28.6275) -> (21.2756, 28.6624) centre (21.8372, 28.1997) ccw construction
  ellipse E2 centre (21.1987, 28.7295) end of major axis (21.1588, 28.8241) minor radius 0.0993 (21.2011, 28.6273) -> (21.2756, 28.6624) ccw
  line L6 (32.7578, 29.9) -> (32.2662, 29.8999) construction
  line L7 (32.2662, 29.8999) -> (32.2664, 29.0446) construction
  line L8 (32.2664, 29.0446) -> (32.758, 29.0447) construction
  ellipse E3 centre (32.7552, 28.9427) end of major axis (32.8028, 29.0337) minor radius 0.0993 (32.8325, 29.0096) -> (32.758, 29.0447) ccw
  arc A4 (32.8325, 29.0096) -> (33.9556, 29.0098) centre (33.3939, 29.4725) ccw construction
  ellipse E4 centre (34.0325, 28.9428) end of major axis (33.9925, 29.0374) minor radius 0.0993 (34.0301, 29.045) -> (33.9556, 29.0098) ccw
  line L9 (34.0301, 29.045) -> (34.5217, 29.0451) construction
  line L10 (34.5217, 29.0451) -> (34.5215, 29.9004) construction
  line L11 (34.5215, 29.9004) -> (33.9826, 29.9003) construction
  arc A5 (33.9826, 29.9003) -> (32.8323, 29.9352) centre (33.3939, 29.4725) ccw construction
  ellipse E5 centre (32.7554, 30.0022) end of major axis (32.7154, 30.0969) minor radius 0.0993 (32.7578, 29.9) -> (32.8323, 29.9352) ccw
  line L12 (32.7608, 17.2) -> (32.2692, 17.1999) construction
  line L13 (32.2692, 17.1999) -> (32.2694, 16.3446) construction
  line L14 (32.2694, 16.3446) -> (32.761, 16.3447) construction
  ellipse E6 centre (32.7582, 16.2427) end of major axis (32.8059, 16.3337) minor radius 0.0993 (32.8356, 16.3096) -> (32.761, 16.3447) ccw
  arc A6 (32.8356, 16.3096) -> (33.9586, 16.3098) centre (33.397, 16.7725) ccw construction
  ellipse E7 centre (34.0355, 16.2428) end of major axis (33.9956, 16.3374) minor radius 0.0993 (34.0331, 16.345) -> (33.9586, 16.3098) ccw
  line L15 (34.0331, 16.345) -> (34.5247, 16.3451) construction
  line L16 (34.5247, 16.3451) -> (34.5245, 17.2004) construction
  line L17 (34.5245, 17.2004) -> (33.9856, 17.2003) construction
  arc A7 (33.9856, 17.2003) -> (32.8354, 17.2352) centre (33.397, 16.7725) ccw construction
  ellipse E8 centre (32.7584, 17.3022) end of major axis (32.7185, 17.3969) minor radius 0.0993 (32.7608, 17.2) -> (32.8354, 17.2352) ccw
  line L18 (32.7639, 4.5) -> (32.2723, 4.4999) construction
  line L19 (32.2723, 4.4999) -> (32.2725, 3.6446) construction
  line L20 (32.2725, 3.6446) -> (32.7641, 3.6447) construction
  ellipse E9 centre (32.7613, 3.5427) end of major axis (32.8089, 3.6337) minor radius 0.0993 (32.8386, 3.6096) -> (32.7641, 3.6447) ccw
  arc A8 (32.8386, 3.6096) -> (33.9616, 3.6098) centre (33.4, 4.0725) ccw construction
  ellipse E10 centre (34.0386, 3.5428) end of major axis (33.9986, 3.6374) minor radius 0.0993 (34.0362, 3.645) -> (33.9616, 3.6098) ccw
  line L21 (34.0362, 3.645) -> (34.5278, 3.6451) construction
  line L22 (34.5278, 3.6451) -> (34.5276, 4.5004) construction
  line L23 (34.5276, 4.5004) -> (33.9886, 4.5003) construction
  arc A9 (33.9886, 4.5003) -> (32.8384, 4.5352) centre (33.4, 4.0725) ccw construction
  ellipse E11 centre (32.7615, 4.6022) end of major axis (32.7215, 4.6969) minor radius 0.0993 (32.7639, 4.5) -> (32.8384, 4.5352) ccw
  circle A10 centre (33.3939, 29.4725) radius 2.54
  circle A11 centre (21.8372, 28.1997) radius 2.54
  circle A12 centre (33.397, 16.7725) radius 2.54
  circle A13 centre (33.4, 4.0725) radius 2.54
  line L24 (37.5933, 33.0302) -> (15.8954, 33.0302)
  line L25 (13.3554, 30.4902) -> (13.3554, 23.6274)
  line L26 (27.9056, -17.5328) -> (37.5933, -17.5328)
  line L27 (40.1333, -14.9928) -> (40.1333, 30.4902)
  circle A14 centre (33.4, 4.0725) radius 3.5577
  circle A15 centre (33.397, 16.7725) radius 3.5577
  circle A16 centre (21.8372, 28.1997) radius 3.5577
  circle A17 centre (33.3939, 29.4725) radius 3.5577
  circle A18 centre (27.9056, -14.9928) radius 2.54
  line L28 (25.3656, -14.9928) -> (25.3656, 18.5474)
  line L29 (22.8256, 21.0874) -> (15.8954, 21.0874)
  arc A19 (37.5933, -17.5328) -> (40.1333, -14.9928) centre (37.5933, -14.9928) ccw
  arc A20 (13.3554, 23.6274) -> (15.8954, 21.0874) centre (15.8954, 23.6274) ccw
  arc A21 (15.8954, 33.0302) -> (13.3554, 30.4902) centre (15.8954, 30.4902) ccw
  arc A22 (40.1333, 30.4902) -> (37.5933, 33.0302) centre (37.5933, 30.4902) ccw
  arc A23 (25.3656, 18.5474) -> (22.8256, 21.0874) centre (22.8256, 18.5474) ccw
  circle A24 centre (20.1878, 21.5954) radius 0.508 construction
  circle A25 centre (33.465, 22.7749) radius 1.905
  circle A26 centre (32.6238, 10.5308) radius 1.905
  circle A27 centre (28.7905, 1.8901) radius 1.27
  circle A28 centre (28.7905, 18.4194) radius 1.27
  circle A29 centre (28.7905, 24.1334) radius 1.27
  line L30 (28.7905, 24.1334) -> (28.7905, 1.8901) construction
  arc A30 (18.2836, 28.3694) -> (18.4188, 27.2141) centre (15.8954, 27.5043) ccw
  dimension "d2" = 5.08
  dimension "d3" = 5.08
  dimension "d4" = 5.08
  dimension "d5" = 5.08
  dimension "d7" = 7.1155
  dimension "d8" = 7.1155
  dimension "d9" = 7.1155
  dimension "d11" = 5.08
  dimension "d12" = 5.08
  dimension "d13" = 7.1155
  dimension "d14" = 2.54
  dimension "d15" = 2.54
  dimension "d16" = 2.54
  dimension "d17" = 2.54
  dimension "d19" = 3.81
  dimension "d20" = 3.81
  dimension "d21" = 2.54
  dimension "d22" = 2.54
  dimension "d23" = 2.54
  measures "d2" diameter of A10
  measures "d3" diameter of A11
  measures "d4" diameter of A12
  measures "d5" diameter of A13
  measures "d7" diameter of A14
  measures "d8" diameter of A15
  measures "d9" diameter of A16
  measures "d11" diameter of A30
  measures "d12" diameter of A18
  measures "d13" diameter of A17
  measures "d14" radius of A19
  measures "d15" radius of A20
  measures "d16" radius of A21
  measures "d17" radius of A23
  measures "d19" diameter of A25
  measures "d20" diameter of A26
  measures "d21" diameter of A27
  measures "d22" diameter of A28
  measures "d23" diameter of A29
extrude "Extrude1" add sketch "Sketch2" against normal blind 1.27 contours A17 | A16 A30 | L24 L25 L26 L27 A18 L28 L29 A19 A20 A21 A22 A23 | A18 | A16 | A14 | A15 | A25 | A26
extrude "Extrude2" add sketch "Sketch2" against normal blind 3.81 contours A16 A30 | L24 L25 L26 L27 A18 L28 L29 A19 A20 A21 A22 A23 | A18 | A25 | A26
extrude "Extrude3" add sketch "Sketch2" against normal blind 7.62 contours A16 A30 | A18 | A25 | A26
equation "d3 = d2"
equation "d4 = d2"
equation "d5 = d2"
equation "d7 = d9"
equation "d8 = d9"
